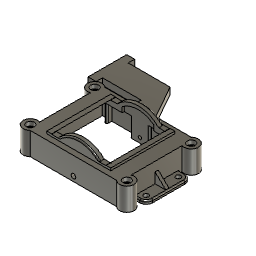
039422-01 MH Roller Assembly Top (Autodesk Fusion 360 archive; units mm, degrees)
design "039422-01 MH Roller Assembly Top" references "039423-01 MH Roller Assembly Bottom"
Autodesk Fusion 360 part; units mm, degrees
note: some values were not read from the file. Set by a fixed rule: which face or edge a step refers to.
(part 1 of 2)
derive "JointPlane" from "039423-01 MH Roller Assembly Bottom v10"
sketch "sketch 195" plane through (0, 0, 0) normal (0, 0, 1) x (1, 0, 0)
  line L0 (42.1069, 33.6931) -> (-42.1068, 33.6931)
  line L1 (-42.1068, 33.6931) -> (-42.1068, -33.6931)
  line L2 (-42.1068, -33.6931) -> (42.1069, -33.6931)
  line L3 (42.1069, -33.6931) -> (42.1069, 33.6931)
  line L4 (42.1069, 33.6931) -> (-42.1068, -33.6931) construction
  line L5 (-42.1068, 33.6931) -> (42.1069, -33.6931) construction
  line L6 (-45.2569, 36.8431) -> (45.2569, 36.8431)
  line L7 (45.2569, 36.8431) -> (45.2569, -36.8431)
  line L8 (45.2569, -36.8431) -> (-45.2569, -36.8431)
  line L9 (-45.2569, -36.8431) -> (-45.2569, 36.8431)
  line L10 (0, 36.8431) -> (0, 33.6931) construction
  line L11 (-42.1068, 0) -> (-45.2569, 0) construction
  line L12 (42.1069, 0) -> (45.2569, 0) construction
  line L13 (0, -33.6931) -> (0, -36.8431) construction
  line L14 (-47.625, 31.75) -> (47.625, 31.75) construction
  line L15 (47.625, 31.75) -> (47.625, -31.75) construction
  line L16 (47.625, -31.75) -> (-47.625, -31.75) construction
  line L17 (-47.625, -31.75) -> (-47.625, 31.75) construction
  line L18 (-47.625, 0) -> (-45.2569, 0) construction
  line L19 (47.625, 0) -> (45.2569, 0) construction
  line L20 (0, 31.75) -> (0, 33.6931) construction
  line L21 (0, -31.75) -> (0, -33.6931) construction
  circle A0 centre (47.625, -31.75) radius 2.7781
  circle A1 centre (47.625, 31.75) radius 2.7781
  circle A2 centre (-47.625, 31.75) radius 2.7781
  circle A3 centre (-47.625, -31.75) radius 2.7781
  circle A4 centre (-47.625, -31.75) radius 3.9688
  circle A5 centre (47.625, -31.75) radius 3.9688
  circle A6 centre (47.625, 31.75) radius 3.9688
  circle A7 centre (-47.625, 31.75) radius 3.9688
  circle A8 centre (-47.625, 31.75) radius 7.1188
  circle A9 centre (-47.625, -31.75) radius 7.1188
  circle A10 centre (47.625, -31.75) radius 7.1188
  circle A11 centre (47.625, 31.75) radius 7.1188
  line L22 (50.8, 15.875) -> (-50.8, 15.875) construction
  line L23 (-50.8, 15.875) -> (-50.8, -15.875) construction
  line L24 (-50.8, -15.875) -> (50.8, -15.875) construction
  line L25 (50.8, -15.875) -> (50.8, 15.875) construction
  line L26 (50.8, 15.875) -> (-50.8, -15.875) construction
  line L27 (-50.8, 15.875) -> (50.8, -15.875) construction
  circle A12 centre (-50.8, -15.875) radius 1.9558
  circle A13 centre (-50.8, 15.875) radius 1.9558
  circle A14 centre (50.8, 15.875) radius 1.9558
  circle A15 centre (50.8, -15.875) radius 1.9558
  circle A16 centre (50.8, 15.875) radius 6.35
  circle A17 centre (50.8, -15.875) radius 6.35
  circle A18 centre (-50.8, -15.875) radius 6.35
  circle A19 centre (-50.8, 15.875) radius 6.35
  line L28 (57.15, 15.875) -> (57.15, -15.875)
  line L29 (-57.15, 15.875) -> (-57.15, -15.875)
  line L30 (-50.8, -22.225) -> (-45.2569, -22.225)
  line L31 (-50.8, 22.225) -> (-45.2569, 22.225)
  line L32 (50.8, 22.225) -> (45.2569, 22.225)
  line L33 (50.8, -22.225) -> (45.2569, -22.225)
  line L34 (-45.2569, 9.525) -> (-50.8, 9.525)
  line L35 (-50.8, -9.525) -> (-45.2569, -9.525)
  line L36 (50.8, 9.525) -> (45.2569, 9.525)
  line L37 (50.8, -9.525) -> (45.2569, -9.525)
  line L38 (-42.1068, -33.6931) -> (-23.3109, -33.6931)
  line L39 (-23.3109, -33.6931) -> (-23.3109, -28.5337)
  line L40 (-23.3109, -28.5337) -> (-42.1068, -28.5337)
  line L41 (-42.1068, -28.5337) -> (-42.1068, -33.6931)
  line L42 (42.1069, -33.6931) -> (23.3109, -33.6931)
  line L43 (23.3109, -33.6931) -> (23.3109, -28.5337)
  line L44 (23.3109, -28.5337) -> (42.1069, -28.5337)
  line L45 (42.1069, -28.5337) -> (42.1069, -33.6931)
  line L46 (42.1069, 33.6931) -> (23.3109, 33.6931)
  line L47 (23.3109, 33.6931) -> (23.3109, 28.5337)
  line L48 (23.3109, 28.5337) -> (42.1069, 28.5337)
  line L49 (42.1069, 28.5337) -> (42.1069, 33.6931)
  line L50 (-42.1068, 33.6931) -> (-23.3108, 33.6931)
  line L51 (-23.3108, 33.6931) -> (-23.3108, 28.5337)
  line L52 (-23.3108, 28.5337) -> (-42.1068, 28.5337)
  line L53 (-42.1068, 28.5337) -> (-42.1068, 33.6931)
extrude "Extrude1" add sketch "sketch 195" along normal blind 22.4155 contours L0 L6 A8 A11 L46 L50 | L0 L3 L6 L7 A6 A11 L46 L49 | L0 L1 L6 L9 A7 A8 L50 L53 | L6 L7 A6 A11 | L6 L9 A7 A8 | L3 L7 A10 A11 A16 A17 | L1 L9 A8 A9 A18 A19 | L7 A1 A6 | L7 A1 A6 | L2 L3 L7 L8 A5 A10 L42 L45 | L9 A2 A7 | L9 A2 A7 | L1 L2 L8 L9 A4 A9 L38 L41 | L7 L8 A5 A10 | L9 A19 | L8 L9 A4 A9 | L7 A16 | L7 A0 A5 | L7 A0 A5 | L2 L8 A9 A10 L38 L42 | L9 A3 A4 | L9 A3 A4 | L7 A17 | L9 A18 picked at (-45.1406, 16.6644) picked at (45.1266, 16.6286) picked at (45.1266, -16.6286) picked at (-45.1406, -16.6644) makes body 1
extrude "Extrude2" add sketch "sketch 195" along normal blind 3.15 contours L9 A19 L31 | L7 A16 L32 | L9 A19 | L7 A16 | L7 A17 L33 | L9 A19 L34 | L9 A18 A19 L29 L34 L35 | L9 A18 L30 | L7 A16 L36 | L7 A16 A17 L28 L36 L37 | L7 A17 | L9 A18 | L7 A17 L37 | L9 A18 L35 picked at (-46.4526, 15.875) picked at (46.4526, 15.875) picked at (46.4526, -15.875) picked at (-46.4526, -15.875) bodies 1
sketch "sketch 867" plane through (0, 0, -3.15) normal (0, 0, -1) x (1, 0, 0)
  line L0 (-57.15, 15.875) -> (-57.15, -15.875)
  arc A0 (-50.8, -9.525) -> (-57.15, -15.875) centre (-50.8, -15.875) ccw
  line L1 (-50.8, -9.525) -> (-45.2569, -9.525)
  line L2 (-45.2569, -9.525) -> (-45.2569, 9.525)
  line L3 (-45.2569, 9.525) -> (-50.8, 9.525)
  arc A1 (-57.15, 15.875) -> (-50.8, 9.525) centre (-50.8, 15.875) ccw
  line L4 (-45.2569, 0) -> (-55.8038, 0) construction
  line L5 (-55.8038, -1.575) -> (-45.2569, -1.575)
  line L6 (-45.2569, -1.575) -> (-45.2569, 1.575)
  line L7 (-45.2569, 1.575) -> (-55.8038, 1.575)
  line L8 (-55.8038, 1.575) -> (-55.8038, -1.575)
  line L9 (-55.8038, -1.575) -> (-45.2569, 1.575) construction
  line L10 (-45.2569, -1.575) -> (-55.8038, 1.575) construction
  line L11 (45.2569, -9.525) -> (50.8, -9.525)
  arc A2 (50.8, -9.525) -> (57.15, -15.875) centre (50.8, -15.875) cw
  line L12 (57.15, -15.875) -> (57.15, 15.875)
  arc A3 (57.15, 15.875) -> (50.8, 9.525) centre (50.8, 15.875) cw
  line L13 (50.8, 9.525) -> (45.2569, 9.525)
  line L14 (45.2569, 9.525) -> (45.2569, -9.525)
  line L15 (45.2569, 0) -> (50.5303, 0) construction
  line L16 (55.8038, 1.575) -> (45.2569, 1.575)
  line L17 (45.2569, 1.575) -> (45.2569, -1.575)
  line L18 (45.2569, -1.575) -> (55.8038, -1.575)
  line L19 (55.8038, -1.575) -> (55.8038, 1.575)
  line L20 (55.8038, 1.575) -> (45.2569, -1.575) construction
  line L21 (45.2569, 1.575) -> (55.8038, -1.575) construction
extrude "Extrude3" add sketch "sketch 867" against normal blind 10.2362 from surface at -6.3 contours L2 L5 L6 L7 L8 | L14 L16 L17 L18 L19 bodies 1
sketch "OutsideSupports" plane through (0, -1.575, 0) normal (0, -1, 0) x (1, 0, 0)
  line L0 (-45.2569, 13.3862) -> (-55.8038, 13.3862)
  line L1 (-55.8038, 13.3862) -> (-55.8038, 3.15)
  line L2 (45.2568, 3.15) -> (55.8038, 3.15)
  line L3 (55.8038, 3.15) -> (55.8038, 13.3862)
  line L4 (55.8038, 13.3862) -> (45.2568, 13.3862)
  line L5 (45.2568, 13.3862) -> (45.2568, 3.15)
  line L6 (45.2568, 13.3862) -> (55.8038, 3.15)
  line L7 (-45.2569, 13.3862) -> (-55.8038, 3.15)
  line L8 (-55.8038, 3.15) -> (-45.2569, 3.15)
  line L9 (-45.2569, 3.15) -> (-45.2569, 13.3862)
  constraint coincident L4.end L5.start
  constraint coincident L2.end L3.start
  constraint coincident L0.start L7.start
  constraint coincident L1.end L7.end
extrude "Extrude4" cut sketch "OutsideSupports" against normal up to surface (3.15 mm away) contours L0 L1 L7 | L3 L4 L6 bodies 1
sketch "TopPlane" plane through (0, 0, 22.4155) normal (0, 0, 1) x (-1, 0, 0)
  line L0 (42.1068, 33.6931) -> (42.1068, -33.6931)
  line L1 (42.1068, -33.6931) -> (-42.1069, -33.6931)
  line L2 (-42.1069, -33.6931) -> (-42.1069, 33.6931)
  line L3 (-42.1069, 33.6931) -> (42.1069, 33.6931)
  arc A0 (-42.6514, 36.8431) -> (-45.2569, 25.0367) centre (-47.625, 31.75) ccw
  line L4 (-45.2569, 25.0367) -> (-45.2569, -25.0367)
  arc A1 (-45.2569, -25.0367) -> (-42.6514, -36.8431) centre (-47.625, -31.75) ccw
  line L5 (-42.6514, -36.8431) -> (42.6514, -36.8431)
  arc A2 (42.6514, -36.8431) -> (45.2569, -25.0367) centre (47.625, -31.75) ccw
  line L6 (45.2569, -25.0367) -> (45.2569, 25.0367)
  arc A3 (45.2569, 25.0367) -> (42.6514, 36.8431) centre (47.625, 31.75) ccw
  line L7 (42.6514, 36.8431) -> (-42.6514, 36.8431)
  line L8 (42.1068, -33.6931) -> (-42.1069, -33.6931)
  line L9 (-42.1069, -33.6931) -> (-42.1069, 33.6931)
  line L10 (-42.1069, 33.6931) -> (42.1068, 33.6931)
  line L11 (42.1068, 33.6931) -> (42.1068, -33.6931)
  line L12 (-26.797, -26.797) -> (26.797, -26.797)
  line L13 (26.797, -26.797) -> (26.797, 26.797)
  line L14 (26.797, 26.797) -> (-26.797, 26.797)
  line L15 (-26.797, 26.797) -> (-26.797, -26.797)
  line L16 (-26.797, -26.797) -> (26.797, 26.797) construction
  line L17 (26.797, -26.797) -> (-26.797, 26.797) construction
  line L18 (31.5595, -31.5595) -> (-31.5595, -31.5595)
  line L19 (-31.5595, -31.5595) -> (-31.5595, 31.5595)
  line L20 (-31.5595, 31.5595) -> (31.5595, 31.5595)
  line L21 (31.5595, 31.5595) -> (31.5595, -31.5595)
  line L22 (31.5595, 0) -> (26.797, 0) construction
  line L23 (-26.797, 0) -> (-31.5595, 0) construction
  line L24 (0, -26.797) -> (0, -31.5595) construction
  line L25 (0, 26.797) -> (0, 31.5595) construction
  line L26 (26.797, -26.797) -> (26.797, -31.5595)
  line L27 (-26.797, -26.797) -> (-26.797, -31.5595)
  line L28 (-26.797, 26.797) -> (-26.797, 31.5595)
  line L29 (26.797, 26.797) -> (26.797, 31.5595)
  circle A4 centre (47.625, 31.75) radius 2.7781
  circle A5 centre (47.625, -31.75) radius 2.7781
  circle A6 centre (-47.625, 31.75) radius 2.7781
  circle A7 centre (-47.625, -31.75) radius 2.7781
  circle A8 centre (-47.625, 31.75) radius 3.937
  circle A9 centre (47.625, 31.75) radius 3.937
  circle A10 centre (47.625, -31.75) radius 3.937
  circle A11 centre (-47.625, -31.75) radius 3.937
  dimension "d59" = 53.594
  dimension "d60" = 53.594
  dimension "d62" = 4.7625
  dimension "d120" = 7.874
  constraint horizontal L8
  constraint vertical L9
  constraint horizontal L10
  constraint vertical L11
  constraint coincident L2.end L3.start
  constraint coincident L0.end L1.start
  constraint horizontal L12
  constraint perpendicular L12 L13
  constraint parallel L12 L14
  constraint parallel L13 L15
  constraint coincident L16 origin
  constraint coincident L17 origin
  constraint horizontal L18
  constraint vertical L19
  constraint horizontal L20
  constraint vertical L21
  constraint midpoint L21 L22.start
  constraint midpoint L13 L22.end
  constraint midpoint L15 L23.start
  constraint midpoint L19 L23.end
  constraint midpoint L12 L24.start
  constraint midpoint L18 L24.end
  constraint midpoint L14 L25.start
  constraint midpoint L20 L25.end
  constraint equal L22 L24
  constraint vertical L24
  constraint horizontal L22
  constraint coincident L18 L26.end
  constraint perpendicular L18 L26
  constraint coincident L18 L27.end
  constraint perpendicular L18 L27
  constraint coincident L20 L28.end
  constraint perpendicular L20 L28
  constraint coincident L20 L29.end
  constraint perpendicular L20 L29
  constraint concentric A0 A8
  constraint concentric A3 A9
  constraint concentric A2 A10
  constraint concentric A1 A11
  constraint equal A8 A9
  constraint equal A9 A10
  constraint equal A10 A11
  measures "d59" distance of L12.end L13.end
  measures "d60" distance of L12.start L12.end
  measures "d62" distance of L22.start L22.end
  measures "d120" diameter of A8
extrude "Extrude5" add sketch "TopPlane" against normal blind 3.15 contours L0 L1 L2 L3 L8 L9 L10 L11 | L15 L18 L19 L20 L27 L28 | L12 L18 L26 L27 | L13 L18 L20 L21 L26 L29 | L14 L20 L28 L29 bodies 1
extrude "Extrude6" add sketch "TopPlane" along normal blind 2.3813 contours L15 L18 L19 L20 L27 L28 | L13 L18 L20 L21 L26 L29 bodies 1
fillet "Fillet1" radius 1.27 5 edges at (48.0284, -22.225, 3.15) (55.2901, -20.3651, 3.15) (57.15, 0, 3.15) (55.2901, 20.3651, 3.15) (48.0284, 22.225, 3.15) on bodies 1
fillet "Fillet1" radius 1.27 5 edges at (-48.0284, 22.225, 3.15) (-55.2901, 20.3651, 3.15) (-57.15, 0, 3.15) (-55.2901, -20.3651, 3.15) (-48.0284, -22.225, 3.15) on bodies 1
extrude "Extrude7" add sketch "TopPlane" along normal blind 1.9844 contours L12 L18 L26 L27 | L14 L20 L28 L29 bodies 1
sketch "FrontOuterPegHole" plane through (0, -36.8431, 0) normal (0, -1, 0) x (1, 0, 0)
  line L0 (-42.6514, 0) -> (42.6514, 0)
  line L1 (42.6514, 0) -> (42.6514, 22.4155)
  line L2 (42.6514, 22.4155) -> (-42.6514, 22.4155)
  line L3 (-42.6514, 22.4155) -> (-42.6514, 0)
  line L4 (0, 0) -> (0, 4.7244) construction
  circle A0 centre (0, 4.7244) radius 2.3241
  dimension "d76" = 4.6482
  dimension "d78" = 4.7244
  constraint coincident L4.start origin
  constraint perpendicular L0 L4
  constraint coincident L4.end A0.centre
  measures "d76" diameter of A0
  measures "d78" distance of L4.start L4.end
sketch "PinchGuardReferenceCircle" plane through (0, -31.5595, 0) normal (0, -1, 0) x (1, 0, 0)
  line L0 (-31.5595, 22.4155) -> (31.5595, 22.4155)
  line L1 (31.5595, 22.4155) -> (31.5595, 24.7967)
  line L2 (31.5595, 24.7967) -> (26.797, 24.7967)
  line L3 (26.797, 24.7967) -> (26.797, 24.3999)
  line L4 (26.797, 24.3999) -> (-26.797, 24.3999)
  line L5 (-26.797, 24.3999) -> (-26.797, 24.7967)
  line L6 (-26.797, 24.7967) -> (-31.5595, 24.7967)
  line L7 (-31.5595, 24.7967) -> (-31.5595, 22.4155)
  circle A0 centre (0, 4.7244) radius 28.3591
  point P0 (0, 4.7244)
  dimension "d80" = 56.7182
  constraint coincident P0 A0.centre
  measures "d80" diameter of A0
extrude "Extrude8" add sketch "PinchGuardReferenceCircle" against normal up to surface (4.7625 mm away) contours L4 A0 bodies 1
extrude "Extrude9" add sketch "PinchGuardReferenceCircle" against normal up to surface (4.7625 mm away) from surface at -58.3565 contours L4 A0 bodies 1
fillet "Fillet2" radius 1.27 2 edges at (0, 31.5595, 33.0835) (0, -31.5595, 33.0835) on bodies 1
sketch "RearInnerPinchGuard" plane through (0, 26.797, 0) normal (0, -1, 0) x (1, 0, 0)
  line L0 (-26.797, 24.3999) -> (-26.797, 19.2655)
  line L1 (-26.797, 19.2655) -> (26.797, 19.2655)
  line L2 (26.797, 19.2655) -> (26.797, 24.3999)
  line L3 (26.797, 24.3999) -> (20.4234, 24.3999)
  arc A0 (20.4234, 24.3999) -> (-20.4234, 24.3999) centre (0, 4.7244) ccw
  line L4 (-20.4234, 24.3999) -> (-26.797, 24.3999)
  circle A1 centre (0, 4.7244) radius 25.1206
  circle A2 centre (0, 4.7244) radius 28.3591
  line L5 (26.797, 24.3999) -> (-26.797, 24.3999)
  line L6 (-15.6179, 24.3999) -> (-15.6179, 19.2655)
  line L7 (15.6179, 24.3999) -> (15.6179, 19.2655)
  line L8 (-15.6179, 19.2655) -> (15.6179, 19.2655)
  point P0 (-15.6179, 24.3999)
  point P1 (15.6179, 24.3999)
  dimension "d90" = 3.2385
  constraint concentric A0 A1
  constraint coincident A1 P0
  constraint coincident P0 L5
  constraint coincident A1 P1
  constraint coincident L5 P1
  constraint coincident P0 L6.start
  constraint coincident L1 L6.end
  constraint perpendicular L1 L6
  constraint coincident P1 L7.start
  constraint coincident L1 L7.end
  constraint perpendicular L1 L7
  measures "d90" distance of A1 A2
sketch "FrontInnerPinchGuard" plane through (0, -26.797, 0) normal (0, 1, 0) x (-1, 0, 0)
  line L0 (-26.797, 24.3999) -> (-26.797, 19.2655)
  line L1 (-26.797, 19.2655) -> (26.797, 19.2655)
  line L2 (26.797, 19.2655) -> (26.797, 24.3999)
  line L3 (26.797, 24.3999) -> (20.4234, 24.3999)
  arc A0 (20.4234, 24.3999) -> (-20.4234, 24.3999) centre (0, 4.7244) ccw
  line L4 (-20.4234, 24.3999) -> (-26.797, 24.3999)
  circle A1 centre (0, 4.7244) radius 25.1206
  line L5 (-15.6179, 24.3999) -> (-15.6179, 19.2655)
  line L6 (15.6179, 24.3999) -> (15.6179, 19.2655)
  line L7 (15.6179, 19.2655) -> (-15.6179, 19.2655)
extrude "Extrude10" cut sketch "FrontInnerPinchGuard" against normal blind 1.9844 contours L1 A1 L5 L6 L7 bodies 1
extrude "Extrude11" cut sketch "RearInnerPinchGuard" against normal blind 1.9844 contours A1 L5 | L1 L5 L6 L7 L8 bodies 1
sketch "PegFlapsAndInnerSupportBase" plane through (0, 0, 19.2655) normal (0, 0, -1) x (1, 0, 0)
  line L0 (15.6179, -26.797) -> (15.6179, -28.7814)
  line L1 (15.6179, -28.7814) -> (-15.6179, -28.7814)
  line L2 (-15.6179, -28.7814) -> (-15.6179, -26.797)
  line L3 (-15.6179, -26.797) -> (-26.797, -26.797)
  line L4 (-26.797, -26.797) -> (-26.797, 26.797)
  line L5 (-26.797, 26.797) -> (-15.6179, 26.797)
  line L6 (-15.6179, 26.797) -> (-15.6179, 28.7814)
  line L7 (-15.6179, 28.7814) -> (15.6179, 28.7814)
  line L8 (15.6179, 28.7814) -> (15.6179, 26.797)
  line L9 (15.6179, 26.797) -> (26.797, 26.797)
  line L10 (26.797, 26.797) -> (26.797, -26.797)
  line L11 (26.797, -26.797) -> (15.6179, -26.797)
  line L12 (42.1069, 33.6931) -> (-42.1068, 33.6931)
  line L13 (-42.1068, 33.6931) -> (-42.1068, -33.6931)
  line L14 (-42.1068, -33.6931) -> (42.1069, -33.6931)
  line L15 (42.1069, -33.6931) -> (42.1069, 33.6931)
  line L16 (-9.525, -31.9564) -> (9.525, -31.9564)
  line L17 (9.525, -31.9564) -> (9.525, -28.7814)
  line L18 (9.525, -28.7814) -> (-9.525, -28.7814)
  line L19 (-9.525, -28.7814) -> (-9.525, -31.9564)
  line L20 (-9.525, -31.9564) -> (9.525, -28.7814) construction
  line L21 (9.525, -31.9564) -> (-9.525, -28.7814) construction
  line L22 (0, -30.3689) -> (0, 0) construction
  line L23 (-9.525, 28.7814) -> (-9.525, 31.9564)
  line L24 (0, 30.3689) -> (0, 0) construction
  line L25 (9.525, 28.7814) -> (-9.525, 31.9564) construction
  line L26 (9.525, 31.9564) -> (9.525, 28.7814)
  line L27 (9.525, 28.7814) -> (-9.525, 28.7814)
  line L28 (-9.525, 31.9564) -> (9.525, 31.9564)
  line L29 (-9.525, 28.7814) -> (9.525, 31.9564) construction
  line L30 (-50.8, 15.875) -> (50.8, 15.875) construction
  line L31 (50.8, -15.875) -> (-50.8, -15.875) construction
  line L32 (-26.797, 17.45) -> (-42.1068, 17.45)
  line L33 (-42.1068, 17.45) -> (-42.1068, 14.3)
  line L34 (-42.1068, 14.3) -> (-26.797, 14.3)
  line L35 (-26.797, 14.3) -> (-26.797, 17.45)
  line L36 (-26.797, 17.45) -> (-42.1068, 14.3) construction
  line L37 (-42.1068, 17.45) -> (-26.797, 14.3) construction
  line L38 (42.1069, 17.45) -> (26.797, 17.45)
  line L39 (26.797, 17.45) -> (26.797, 14.3)
  line L40 (26.797, 14.3) -> (42.1069, 14.3)
  line L41 (42.1069, 14.3) -> (42.1069, 17.45)
  line L42 (42.1069, 17.45) -> (26.797, 14.3) construction
  line L43 (26.797, 17.45) -> (42.1069, 14.3) construction
  line L44 (-42.1068, -33.6931) -> (-42.1068, 33.6931)
  line L45 (-26.797, -26.797) -> (-26.797, 26.797)
  line L46 (42.1069, 33.6931) -> (42.1069, -33.6931)
  line L47 (26.797, 26.797) -> (26.797, -26.797)
  line L48 (-26.797, -14.3) -> (-42.1068, -14.3)
  line L49 (-42.1068, -14.3) -> (-42.1068, -17.45)
  line L50 (-42.1068, -17.45) -> (-26.797, -17.45)
  line L51 (-26.797, -17.45) -> (-26.797, -14.3)
  line L52 (-26.797, -14.3) -> (-42.1068, -17.45) construction
  line L53 (-42.1068, -14.3) -> (-26.797, -17.45) construction
  line L54 (26.797, -14.3) -> (42.1069, -14.3)
  line L55 (42.1069, -14.3) -> (42.1069, -17.45)
  line L56 (42.1069, -17.45) -> (26.797, -17.45)
  line L57 (26.797, -17.45) -> (26.797, -14.3)
  line L58 (26.797, -14.3) -> (42.1069, -17.45) construction
  line L59 (42.1069, -14.3) -> (26.797, -17.45) construction
  line L60 (-35.7568, -33.6931) -> (-32.6068, -33.6931)
  line L61 (-32.6068, -33.6931) -> (-32.6068, -28.9306)
  line L62 (-32.6068, -28.9306) -> (-35.7568, -28.9306)
  line L63 (-35.7568, -28.9306) -> (-35.7568, -33.6931)
  line L64 (32.6069, -33.6931) -> (35.7569, -33.6931)
  line L65 (35.7569, -33.6931) -> (35.7569, -28.9306)
  line L66 (35.7569, -28.9306) -> (32.6069, -28.9306)
  line L67 (32.6069, -28.9306) -> (32.6069, -33.6931)
  line L68 (35.7569, 33.6931) -> (32.6069, 33.6931)
  line L69 (32.6069, 33.6931) -> (32.6069, 28.9306)
  line L70 (32.6069, 28.9306) -> (35.7569, 28.9306)
  line L71 (35.7569, 28.9306) -> (35.7569, 33.6931)
  line L72 (-32.6068, 33.6931) -> (-35.7568, 33.6931)
  line L73 (-35.7568, 33.6931) -> (-35.7568, 28.9306)
  line L74 (-35.7568, 28.9306) -> (-32.6068, 28.9306)
  line L75 (-32.6068, 28.9306) -> (-32.6068, 33.6931)
  line L76 (42.1069, -33.6931) -> (35.7569, -33.6931) construction
  line L77 (-35.7568, -33.6931) -> (-42.1068, -33.6931) construction
  line L78 (-35.7568, 33.6931) -> (-42.1068, 33.6931) construction
  line L79 (35.7569, 33.6931) -> (42.1069, 33.6931) construction
  point P0 (0, -30.3689)
  point P1 (0, 30.3689)
  point P2 (-34.4519, 15.875)
  point P3 (34.4519, 15.875)
  point P4 (-34.4519, -15.875)
  point P5 (34.4519, -15.875)
  dimension "d98" = 19.05
  dimension "d99" = 3.175
  dimension "d100" = 19.05
  dimension "d101" = 3.175
  dimension "d123" = 3.15
  dimension "d148" = 3.15
  dimension "d149" = 3.15
  dimension "d150" = 3.15
  dimension "d151" = 3.15
  dimension "d153" = 4.7625
  dimension "d154" = 6.35
  constraint horizontal L16
  constraint perpendicular L16 L17
  constraint parallel L16 L18
  constraint parallel L17 L19
  constraint coincident L20 P0
  constraint coincident L21 P0
  constraint coincident P0 L22.start
  constraint coincident L22.end L24.end
  constraint vertical L22
  constraint collinear L1 L18
  constraint perpendicular L23 L27
  constraint parallel L27 L28
  constraint parallel L23 L26
  constraint coincident P1 L25
  constraint coincident P1 L29
  constraint coincident P1 L24.start
  constraint collinear L7 L27
  constraint vertical L24
  constraint horizontal L32
  constraint perpendicular L32 L33
  constraint parallel L32 L34
  constraint parallel L33 L35
  constraint coincident L36 P2
  constraint coincident L37 P2
  constraint coincident L30 P2
  constraint horizontal L38
  constraint perpendicular L38 L39
  constraint parallel L38 L40
  constraint parallel L39 L41
  constraint coincident L42 P3
  constraint coincident L43 P3
  constraint coincident L30 P3
  constraint collinear L33 L44
  constraint collinear L35 L45
  constraint collinear L41 L46
  constraint collinear L39 L47
  constraint equal L35 L39
  constraint horizontal L48
  constraint perpendicular L48 L49
  constraint parallel L48 L50
  constraint parallel L49 L51
  constraint coincident L52 P4
  constraint coincident L53 P4
  constraint coincident L31 P4
  constraint horizontal L54
  constraint perpendicular L54 L55
  constraint parallel L54 L56
  constraint parallel L55 L57
  constraint coincident L58 P5
  constraint coincident L59 P5
  constraint coincident L31 P5
  constraint equal L51 L57
  constraint equal L35 L51
  constraint collinear L44 L49
  constraint collinear L45 L51
  constraint collinear L46 L55
  constraint collinear L47 L57
  constraint horizontal L60
  constraint vertical L61
  constraint horizontal L62
  constraint vertical L63
  constraint coincident L14 L60.start
  constraint horizontal L64
  constraint vertical L65
  constraint horizontal L66
  constraint vertical L67
  constraint coincident L14 L64.start
  constraint horizontal L68
  constraint vertical L69
  constraint horizontal L70
  constraint vertical L71
  constraint coincident L12 L68.start
  constraint horizontal L72
  constraint vertical L73
  constraint horizontal L74
  constraint vertical L75
  constraint coincident L12 L72.start
  constraint equal L69 L73
  constraint equal L67 L69
  constraint equal L63 L67
  constraint coincident L14.end L15.start
  constraint coincident L13.end L14.start
  constraint perpendicular L13 L77
  constraint coincident L12.end L13.start
  constraint perpendicular L13 L78
  constraint coincident L12.start L15.end
  constraint perpendicular L46 L79
  constraint equal L78 L79
  constraint equal L76 L79
  constraint equal L76 L77
  measures "d98" distance of L17.end L18.end
  measures "d99" distance of L16.start L18.end
  measures "d100" distance of L26.start L23.end
  measures "d101" distance of L25.start L26.start
  measures "d123" distance of L32.start L34.end
  measures "d148" distance of L60.start L60.end
  measures "d149" distance of L64.start L64.end
  measures "d150" distance of L68.start L68.end
  measures "d151" distance of L72.start L72.end
  measures "d153" distance of L72.end L73.end
  measures "d154" distance of L60.start L13.end
extrude "Extrude12" add sketch "PegFlapsAndInnerSupportBase" along normal up to surface (19.2655 mm away) contours L1 L16 L17 L18 L19 | L14 L64 L65 L66 L67 | L14 L60 L61 L62 L63 | L12 L68 L69 L70 L71 | L7 L23 L26 L27 L28 | L12 L72 L73 L74 L75 bodies 1
fillet "Fillet3" radius 1.27 8 edges at (-9.525, 28.7814, 9.6327) (-9.525, 31.9564, 9.6327) (9.525, 28.7814, 9.6327) (-9.525, -31.9564, 9.6327) (-9.525, -28.7814, 9.6327) (9.525, -31.9564, 9.6327) (9.525, -28.7814, 9.6327) (9.525, 31.9564, 9.6327) on bodies 1
fillet "Fillet3" radius 1.27 8 edges at (-35.7568, -28.9306, 9.6327) (-32.6068, -28.9306, 9.6327) (32.6069, -28.9306, 9.6327) (35.7569, -28.9306, 9.6327) (-35.7568, 28.9306, 9.6327) (-32.6068, 28.9306, 9.6327) (32.6069, 28.9306, 9.6327) (35.7569, 28.9306, 9.6327) on bodies 1
sketch "RearOuterPegHole" plane through (0, 36.8431, 0) normal (0, 1, 0) x (-1, 0, 0)
  line L0 (-42.6514, 0) -> (42.6514, 0)
  line L1 (42.6514, 0) -> (42.6514, 22.4155)
  line L2 (42.6514, 22.4155) -> (-42.6514, 22.4155)
  line L3 (-42.6514, 22.4155) -> (-42.6514, 0)
  circle A0 centre (0, 4.7244) radius 2.3241
  circle A1 centre (0, 4.7244) radius 2.3241
  point P0 (0, 4.7244)
  constraint concentric A0 A1
  constraint equal A0 A1
extrude "Extrude13" cut sketch "RearOuterPegHole" against normal up to surface (3.15 mm away) contours A0 A1 bodies 1
extrude "Extrude14" cut sketch "FrontOuterPegHole" against normal up to surface (3.15 mm away) contours A0 bodies 1
sketch "InnerPegHoles" plane through (0, -31.9564, 0) normal (0, -1, 0) x (1, 0, 0)
  line L0 (8.255, 0) -> (8.255, 19.2655)
  line L1 (8.255, 19.2655) -> (-8.255, 19.2655)
  line L2 (-8.255, 19.2655) -> (-8.255, 0)
  line L3 (-8.255, 0) -> (8.255, 0)
  circle A0 centre (0, 4.7244) radius 1.632
  point P0 (0, 4.7244)
  dimension "d111" = 3.2639
  constraint coincident P0 A0.centre
  measures "d111" diameter of A0
extrude "Extrude15" cut sketch "InnerPegHoles" against normal up to surface (63.9127 mm away) contours A0 bodies 1
sketch "JointCounterbores" plane through (0, 0, 0) normal (0, 0, -1) x (1, 0, 0)
  circle A0 centre (50.8, 15.875) radius 1.9558
  circle A1 centre (50.8, -15.875) radius 1.9558
  circle A2 centre (-50.8, 15.875) radius 1.9558
  circle A3 centre (-50.8, -15.875) radius 1.9558
  circle A4 centre (-47.625, 31.75) radius 2.7781
  circle A5 centre (-47.625, -31.75) radius 2.7781
  line L0 (-42.1068, -33.6931) -> (-42.1068, 33.6931)
  line L1 (-42.1068, 33.6931) -> (-35.7568, 33.6931)
  line L2 (42.1069, 33.6931) -> (42.1069, -33.6931)
  line L3 (42.1069, -33.6931) -> (35.7569, -33.6931)
  circle A6 centre (47.625, 31.75) radius 2.7781
  circle A7 centre (47.625, -31.75) radius 2.7781
  arc A8 (45.2569, 25.0367) -> (42.6514, 36.8431) centre (47.625, 31.75) ccw
  line L4 (42.6514, 36.8431) -> (-42.6514, 36.8431)
  arc A9 (-42.6514, 36.8431) -> (-45.2569, 25.0367) centre (-47.625, 31.75) ccw
  line L5 (-45.2569, 25.0367) -> (-45.2569, 22.225)
  line L6 (-45.2569, 22.225) -> (-50.8, 22.225)
  arc A10 (-50.8, 22.225) -> (-57.15, 15.875) centre (-50.8, 15.875) ccw
  line L7 (-57.15, 15.875) -> (-57.15, -15.875)
  arc A11 (-57.15, -15.875) -> (-50.8, -22.225) centre (-50.8, -15.875) ccw
  line L8 (-50.8, -22.225) -> (-45.2569, -22.225)
  line L9 (-45.2569, -22.225) -> (-45.2569, -25.0367)
  arc A12 (-45.2569, -25.0367) -> (-42.6514, -36.8431) centre (-47.625, -31.75) ccw
  line L10 (-42.6514, -36.8431) -> (42.6514, -36.8431)
  arc A13 (42.6514, -36.8431) -> (45.2569, -25.0367) centre (47.625, -31.75) ccw
  line L11 (45.2569, -25.0367) -> (45.2569, -22.225)
  line L12 (45.2569, -22.225) -> (50.8, -22.225)
  arc A14 (50.8, -22.225) -> (57.15, -15.875) centre (50.8, -15.875) ccw
  line L13 (57.15, -15.875) -> (57.15, 15.875)
  arc A15 (57.15, 15.875) -> (50.8, 22.225) centre (50.8, 15.875) ccw
  line L14 (50.8, 22.225) -> (45.2569, 22.225)
  line L15 (45.2569, 22.225) -> (45.2569, 25.0367)
  circle A16 centre (-47.625, 31.75) radius 4.0323
  circle A17 centre (47.625, 31.75) radius 4.0323
  circle A18 centre (47.625, -31.75) radius 4.0323
  circle A19 centre (-47.625, -31.75) radius 4.0323
  line L16 (-35.7568, 33.6931) -> (-35.7568, 30.2006)
  line L17 (-34.4868, 28.9306) -> (-33.8768, 28.9306)
  line L18 (-32.6068, 30.2006) -> (-32.6068, 33.6931)
  line L19 (-32.6068, 33.6931) -> (32.6069, 33.6931)
  line L20 (32.6069, 33.6931) -> (32.6069, 30.2006)
  line L21 (33.8769, 28.9306) -> (34.4869, 28.9306)
  line L22 (35.7569, 30.2006) -> (35.7569, 33.6931)
  line L23 (35.7569, 33.6931) -> (42.1069, 33.6931)
  line L24 (35.7569, -33.6931) -> (35.7569, -30.2006)
  line L25 (34.4869, -28.9306) -> (33.8769, -28.9306)
  line L26 (32.6069, -30.2006) -> (32.6069, -33.6931)
  line L27 (32.6069, -33.6931) -> (-32.6068, -33.6931)
  line L28 (-32.6068, -33.6931) -> (-32.6068, -30.2006)
  line L29 (-33.8768, -28.9306) -> (-34.4868, -28.9306)
  line L30 (-35.7568, -30.2006) -> (-35.7568, -33.6931)
  line L31 (-35.7568, -33.6931) -> (-42.1068, -33.6931)
  arc A20 (35.7569, -30.2006) -> (34.4869, -28.9306) centre (34.4869, -30.2006) ccw
  arc A21 (33.8769, -28.9306) -> (32.6069, -30.2006) centre (33.8769, -30.2006) ccw
  arc A22 (-32.6068, -30.2006) -> (-33.8768, -28.9306) centre (-33.8768, -30.2006) ccw
  arc A23 (-34.4868, -28.9306) -> (-35.7568, -30.2006) centre (-34.4868, -30.2006) ccw
  arc A24 (-35.7569, 30.2006) -> (-34.4868, 28.9306) centre (-34.4868, 30.2006) ccw
  arc A25 (-33.8768, 28.9306) -> (-32.6068, 30.2006) centre (-33.8768, 30.2006) ccw
  arc A26 (32.6069, 30.2006) -> (33.8769, 28.9306) centre (33.8769, 30.2006) ccw
  arc A27 (34.4869, 28.9306) -> (35.7569, 30.2006) centre (34.4869, 30.2006) ccw
  dimension "d117" = 8.0645
  constraint concentric A4 A16
  constraint concentric A6 A17
  constraint concentric A7 A18
  constraint concentric A5 A19
  constraint equal A16 A17
  constraint equal A17 A18
  constraint equal A18 A19
  measures "d117" diameter of A16
extrude "Extrude16" cut sketch "JointCounterbores" against normal blind 4.064 contours A16 | A17 | A18 | A19 bodies 1
extrude "Extrude17" cut sketch "TopPlane" against normal blind 4.064 contours A8 | A9 | A10 | A11 bodies 1
extrude "Extrude18" add sketch "PegFlapsAndInnerSupportBase" along normal blind 9.7536 contours L10 L15 L46 L47 L54 L55 L56 L57 | L10 L15 L38 L39 L40 L41 L46 L47 | L4 L13 L44 L45 L48 L49 L50 L51 | L4 L13 L32 L33 L34 L35 L44 L45 bodies 1
sketch "InnerSupports" plane through (0, 17.45, 0) normal (0, 1, 0) x (-1, 0, 0)
  line L0 (42.1068, 19.2655) -> (26.797, 19.2655)
  line L1 (26.797, 19.2655) -> (26.797, 9.5119)
  line L2 (26.797, 9.5119) -> (42.1068, 9.5119)
  line L3 (42.1068, 9.5119) -> (42.1068, 19.2655)
  line L4 (-26.797, 19.2655) -> (-42.1069, 19.2655)
  line L5 (-42.1069, 19.2655) -> (-42.1069, 9.5119)
  line L6 (-42.1069, 9.5119) -> (-26.797, 9.5119)
  line L7 (-26.797, 9.5119) -> (-26.797, 19.2655)
  line L8 (-26.797, 24.7967) -> (-31.5595, 24.7967)
  line L9 (-31.5595, 24.7967) -> (-26.797, 24.7967)
  line L10 (26.797, 24.7967) -> (31.5595, 24.7967)
  line L11 (31.5595, 24.7967) -> (26.797, 24.7967)
  line L12 (-26.797, 24.7967) -> (-26.797, 9.5119)
  line L13 (26.797, 9.5119) -> (26.797, 24.7967)
  line L14 (-42.1069, 9.5119) -> (-32.9477, 19.2655)
  line L15 (-42.1069, 9.5119) -> (-35.0981, 9.5119) construction
  line L16 (42.1068, 9.5119) -> (32.9477, 19.2655)
  line L17 (42.1068, 9.5119) -> (33.1786, 9.5119) construction
  line L18 (26.797, 24.7967) -> (42.1068, 9.9564)
  line L19 (-26.797, 24.7967) -> (-42.1069, 9.9564)
  line L20 (42.1068, 9.5119) -> (42.1068, 9.9564) construction
  line L21 (32.9477, 19.2655) -> (32.5032, 19.2655) construction
  line L22 (-42.1069, 9.5119) -> (-42.1069, 9.9564) construction
  line L23 (-32.9477, 19.2655) -> (-32.5032, 19.2655) construction
  dimension "d147" = 0.4445
  constraint coincident L8.start L9.end
  constraint coincident L6.end L7.start
  constraint coincident L1.end L2.start
  constraint coincident L10.start L11.end
  constraint horizontal L15
  constraint coincident L5.end L6.start
  constraint coincident L4 L14.end
  constraint horizontal L17
  constraint coincident L2.end L3.start
  constraint coincident L0 L16.end
  constraint coincident L3 L18.end
  constraint coincident L5 L19.end
  constraint coincident L18 L21.end
  constraint coincident L0 L21.end
  constraint equal L20 L21
  constraint perpendicular L6 L22
  constraint coincident L19 L23.end
  constraint coincident L4 L23.end
  constraint equal L22 L23
  constraint equal L21 L23
  measures "d147" distance of L2.end L18.end
extrude "Extrude19" cut sketch "InnerSupports" along normal up to surface (9.347 mm away) and the other way up to surface (44.247 mm away) contours L0 L16 L18 | L0 L1 L2 L13 L16 L18 | L0 L13 L18 | L4 L14 L19 | L4 L12 L19 | L4 L6 L7 L12 L14 L19 bodies 1
ref_plane "WorkPlane1" through (-61.9125, 58.547, -33.3375) normal (1, 0, 0) x (0, 1, 0)
sketch "EncodingArmDistance" plane through (-61.9125, 0, 0) normal (1, 0, 0) x (0, 1, 0)
  line L0 (77.597, -33.3375) -> (39.497, -33.3375) construction
  line L1 (39.497, -33.3375) -> (39.497, 20.3708) construction
  line L2 (39.497, 20.3708) -> (77.597, 20.3708) construction
  line L3 (77.597, 20.3708) -> (77.597, -33.3375) construction
  point P0 (39.497, -33.3375)
  point P1 (58.547, -33.3375)
  point P2 (77.597, -33.3375)
  dimension "d132" = 53.7083
  constraint horizontal L0
  constraint vertical L1
  constraint horizontal L2
  constraint vertical L3
  constraint coincident P2 L0.start
  constraint coincident P0 L0.end
  measures "d132" distance of P2 L2.end
ref_plane "WorkPlane2" through (-61.9125, 58.547, 20.3708) normal (0, 0, 1) x (0, 1, 0)
sketch "UpperEncodingArm" plane through (0, 0, 20.3708) normal (0, 0, 1) x (1, 0, 0)
  line L0 (-12.725, 71.247) -> (6.5659, 36.8431)
  line L1 (-12.725, 65.6292) -> (3.4159, 36.8431)
  line L2 (-15.875, 71.247) -> (-53.975, 71.247)
  line L3 (-53.975, 68.097) -> (-15.875, 68.097)
  line L4 (-53.975, 48.997) -> (-15.875, 48.997)
  line L5 (-53.975, 45.847) -> (-15.875, 45.847)
  line L6 (-15.875, 45.847) -> (-15.875, 71.247)
  line L7 (-15.875, 36.8431) -> (-15.875, 71.247)
  line L8 (-12.725, 36.8431) -> (-12.725, 65.6292)
  line L9 (-53.975, 77.597) -> (-53.975, 39.497)
  line L10 (-57.1119, 74.0251) -> (-57.1119, 43.0689)
  line L11 (-58.7756, 43.0689) -> (-58.7756, 74.0251)
  line L12 (-12.725, 65.6292) -> (-12.725, 68.097)
  line L13 (-12.725, 68.097) -> (-15.875, 68.097)
  line L14 (-15.875, 71.247) -> (-12.725, 71.247)
  line L15 (-53.975, 39.497) -> (-61.9125, 39.497)
  line L16 (-61.9125, 77.597) -> (-53.975, 77.597)
  line L17 (-61.9125, 39.497) -> (-61.9125, 77.597)
  line L18 (-58.7756, 74.0251) -> (-57.1119, 74.0251)
  line L19 (-57.1119, 43.0689) -> (-58.7756, 43.0689)
  line L20 (-57.9438, 43.0689) -> (-57.9438, 39.497)
  line L21 (-57.9438, 74.0251) -> (-57.9438, 77.597)
  line L22 (-57.1119, 58.547) -> (-53.975, 58.547)
  line L23 (-58.7756, 58.547) -> (-61.9125, 58.547)
  line L24 (-47.625, 31.75) -> (-47.625, 71.247)
  line L25 (-12.725, 36.8431) -> (-15.875, 36.8431)
  line L26 (6.5659, 36.8431) -> (3.4159, 36.8431)
  line L27 (3.4159, 36.8431) -> (-12.725, 36.8431)
  constraint coincident L8.start L25.start
  constraint coincident L7.start L25.end
  constraint coincident L0.end L26.start
  constraint coincident L1.end L26.end
extrude "Extrude20" add sketch "UpperEncodingArm" against normal blind 2.9083 contours L1 L8 L27 | L3 L4 L6 L7 L24 | L3 L4 L9 L24 | L10 L11 L18 L19 bodies 1 makes body 2 at (-28.575, 55.3637, 20.3708) makes body 3 at (-57.1119, 63.7064, 19.4014)
extrude "Extrude21" add sketch "UpperEncodingArm" against normal blind 6.5532 contours L0 L1 L6 L7 L12 L13 L14 L26 | L2 L3 L6 L7 L24 | L2 L3 L9 L24 | L9 L10 L16 L18 L21 L22 | L4 L5 L6 L7 L24 | L4 L5 L9 L24 | L11 L16 L17 L18 L21 L23 | L9 L10 L15 L19 L20 L22 | L11 L15 L17 L19 L20 L23 bodies 1 2 3
extrude "Extrude22" add sketch "UpperEncodingArm" against normal blind 14.0589 contours L6 L7 L8 L12 L13 L25 bodies 1
sketch "UpperEncodingArmSupport" plane through (-15.875, 0, 0) normal (-1, 0, 0) x (0, -1, 0)
  line L0 (-45.847, 20.3708) -> (-45.847, 13.8176)
  line L1 (-45.847, 13.8176) -> (-48.997, 13.8176)
  line L2 (-48.997, 13.8176) -> (-48.997, 17.4625)
  line L3 (-48.997, 17.4625) -> (-68.097, 17.4625)
  line L4 (-68.097, 17.4625) -> (-68.097, 13.8176)
  line L5 (-68.097, 13.8176) -> (-68.097, 6.3119)
  line L6 (-68.097, 6.3119) -> (-36.8431, 6.3119)
  line L7 (-36.8431, 6.3119) -> (-36.8431, 20.3708)
  line L8 (-36.8431, 20.3708) -> (-45.847, 20.3708)
  line L9 (-71.247, 13.8176) -> (-68.097, 13.8176)
  line L10 (-48.997, 13.8176) -> (-45.847, 13.8176)
  line L11 (-36.8431, 6.3119) -> (-68.097, 13.8176)
  constraint coincident L6.end L7.start
  constraint coincident L4.end L5.start
extrude "Extrude23" cut sketch "UpperEncodingArmSupport" against normal up to surface (3.15 mm away) contours L5 L6 L11 bodies 1
sketch "Sketch16" plane through (0, 0, 3.15) normal (0, 0, 1) x (-1, 0, 0)
  line L0 (50.8, 20.955) -> (45.2569, 20.955)
  line L1 (45.2569, 20.955) -> (45.2569, 1.575)
  line L2 (45.2569, 1.575) -> (55.8038, 1.575)
  line L3 (55.8038, 1.575) -> (55.8038, -1.575)
  line L4 (55.8038, -1.575) -> (45.2569, -1.575)
  line L5 (45.2569, -1.575) -> (45.2569, -20.955)
  line L6 (45.2569, -20.955) -> (50.8, -20.955)
  arc A0 (50.8, -20.955) -> (55.88, -15.875) centre (50.8, -15.875) ccw
  line L7 (55.88, -15.875) -> (55.88, 15.875)
  arc A1 (55.88, 15.875) -> (50.8, 20.955) centre (50.8, 15.875) ccw
  circle A2 centre (50.8, -15.875) radius 1.9558
  circle A3 centre (50.8, 15.875) radius 1.9558
  circle A4 centre (50.8, 15.875) radius 1.9558
  circle A5 centre (50.8, -15.875) radius 1.9558
  circle A6 centre (-50.8, -15.875) radius 1.9558
  circle A7 centre (-50.8, 15.875) radius 1.9558
  circle A8 centre (-50.8, 15.875) radius 2.3812
  circle A9 centre (-50.8, -15.875) radius 2.3812
  circle A10 centre (50.8, 15.875) radius 2.3812
  circle A11 centre (50.8, -15.875) radius 2.3812
  dimension "d204" = 4.7625
  constraint concentric A7 A8
  constraint concentric A6 A9
  constraint concentric A4 A10
  constraint concentric A5 A11
  constraint equal A8 A9
  constraint equal A9 A11
  constraint equal A10 A11
  measures "d204" diameter of A8
extrude "Extrude24" cut sketch "Sketch16" against normal up to surface (3.15 mm away) contours A2 A5 | A3 A4 | A6 | A7 | A8 | A9 | A10 | A11 bodies 1
equation "d1 = UpperBodyHeight"
equation "UpperBodyHeight = 0.8825 in"
equation "WallThickness_Ref = 3.15 mm"
equation "MountingWidthCTC_Ref = 3.75 in"
equation "MountingHeightCTC_Ref = 2.5 in"
equation "MountingDiameter_Ref = ( 7 / 32 ) * 1 in"
equation "MountingDowelThickness_Ref = ( 3 / 64 ) * 1 in"
equation "MountingDowelOutsideDiameter_Ref = MountingDiameter_Ref + ( 2 * MountingDowelThickness_Ref )"
equation "MountingOutsideDiameter_Ref = MountingDowelOutsideDiameter_Ref + ( 2 * WallThickness_Ref )"
equation "MatingHoleWidthCTC_Ref = 4 in"
equation "MatingHoleHeightCTC_Ref = 1 1/4\""
equation "MatingHolePassthroughDiameter_Ref = ( 3 / 16 ) * 1 in"
equation "MatingHoleThreadedDiameter_Ref = ( 1 / 8 ) * 1 in"
equation "MatingHoleSupportDiameter_Ref = ( 1 / 2 ) * 1 in"
equation "BodyBottomDepth_Ref = 1 5/16\""
equation "MountingDowelHeight_Ref = ( 1 / 8 ) * 1 in"
equation "MountingDowelClearance_Ref = 0.01 in"
equation "BearingBoxWidth_Ref = ( 13 / 64 ) * 1 in"
equation "BearingBoxLength_Ref = 0.74 in"
equation "BottomCenterHoleDiameter_Ref = ( 3 / 4 ) * 1 in"
equation "BottomCornerHoleDiameter_Ref = ( 3 / 8 ) * 1 in"
equation "BottomCornerHoleWidthCTC_Ref = 2 11/16\""
equation "BottomCornerHoleHeightCTC_Ref = 1 51/64\""
equation "EncoderArmHeight_Ref = 1 in"
equation "EncoderArmLength_Ref = 1 1/2\""
equation "EncoderArmTriangleBase_Ref = 0.8835 in"
equation "PCBHolderWidth_Ref = ( 5 / 16 ) * 1 in"
equation "PCBHolderHeight_Ref = 1 1/2\""
equation "InsideHeight_Ref = 2.6530 in"
equation "PCBWidth_Ref = 0.0655 in"
equation "PCBHeight_Ref = 1 7/32\""
equation "EncoderArmThickness_Ref = 0.258 in"
equation "EncoderArmInsideThickness_Ref = EncoderArmThickness_Ref - 0.1435 in"
equation "EncoderArmSupportHeight_Ref = 0.9685 in"
equation "LightScrewDistanceToEdgeOfInnerCircle_Ref = 1.1285 in"
equation "LightScrewDiameter_Ref = MatingHoleThreadedDiameter_Ref"
equation "BearinBoxReliefWidth_Ref = ( 5 / 8 ) * 1 in"
equation "BearingBoxReliefHeight_Ref = 0.07 in"
equation "InnerSupportHeight_Ref = 0.6940 in"
equation "InnerSupportLenth_Ref = 1 1/4\""
equation "BearingOD_Ref = ( 5 / 8 ) * 1 in"
equation "BearingChannelDepth_Ref = 0.6255 in"
equation "BearingExtraWidth_Ref = ( 1 / 16 ) * 1 in"
equation "BearingExtraDepth_Ref = ( 1 / 32 ) * 1 in"
equation "ShaftOpeningDiameter_Ref = ( 5 / 16 ) * 1 in"
equation "OutsideSupportOffset_Ref = 0.053 in"
equation "OutsideSupportHeight_Ref = 0.6 in"
equation "d49 = WallThickness_Ref"
equation "d51 = -OutsideSupportHeight"
equation "OutsideSupportHeight = 0.4030 in"
equation "TopOpeningHeight = 2.110 in"
equation "TopOpeningWidth = TopOpeningHeight"
equation "d59 = TopOpeningHeight"
equation "d60 = TopOpeningWidth"
equation "TopOpeningBorder = ( 3 / 16 ) * 1 in"
equation "d62 = TopOpeningBorder"
equation "d63 = -WallThickness_Ref"
equation "d65 = TopOpeningBorderThicknessSides"
equation "d68 = Fillet_Ref"
equation "d70 = Fillet_Ref"
equation "TopOpeningBorderThicknessMiddle = TopOpeningBorderThicknessSides - ( ( 1 / 64 ) * 1 in )"
equation "d72 = TopOpeningBorderThicknessMiddle"
equation "TopOpeningBorderThicknessSides = ( ( 3 / 32 ) * 1 ) * 1 in"
equation "PegOutsideDiameter = 0.1830 in"
equation "d76 = PegOutsideDiameter"
equation "PegDistanceFromEdge = ( ( 0.0955 + 0.2765 ) / 2 ) * 1 in"
equation "d78 = PegDistanceFromEdge"
equation "PinchGuardCircleRadius = 1.025 in + ( PegOutsideDiameter / 2 )"
equation "d80 = PinchGuardCircleRadius * 2"
equation "Fillet_Ref = 0.05 in"
equation "d88 = Fillet_Ref"
equation "PinchGuardInnerLip = 0.1275 in"
equation "d90 = PinchGuardInnerLip"
equation "PinchGuardInnerDepth = ( 5 / 64 ) * 1 in"
equation "d92 = -PinchGuardInnerDepth"
equation "d94 = -PinchGuardInnerDepth"
equation "PegFlapWidth = ( 3 / 4 ) * 1 in"
equation "PegFlapThickness = ( 1 / 8 ) * 1 in"
equation "d98 = PegFlapWidth"
equation "d99 = PegFlapThickness"
equation "d100 = PegFlapWidth"
equation "d101 = PegFlapThickness"
equation "d105 = Fillet_Ref"
equation "InnerPegHoleDiameter = 0.1285 in"
equation "d111 = InnerPegHoleDiameter"
equation "JointCounterboreDiameter = 0.3175 in"
equation "TopCounterboreDiameter = 0.31 in"
equation "CounterboreDepth = 0.160 in"
equation "d117 = JointCounterboreDiameter"
equation "d118 = -CounterboreDepth"
equation "d120 = TopCounterboreDiameter"
equation "d121 = -CounterboreDepth"
equation "d123 = WallThickness_Ref"
equation "d124 = InnerSupportHeight"
equation "InnerSupportHeight = 0.384 in"
equation "d132 = EncoderArmOutsideHeight"
equation "EncoderArmOutsideHeight = 2 in + EncoderArmInsideThickness_Ref"
equation "d135 = -EncoderArmInsideThickness_Ref"
equation "d137 = -EncoderArmThickness_Ref"
equation "UpperEncoderArmSupportHeight = 0.5535 in"
equation "d140 = -UpperEncoderArmSupportHeight"
equation "InnerSupportGap = 0.0175 in"
equation "d147 = InnerSupportGap"
equation "d148 = WallThickness_Ref"
equation "d149 = WallThickness_Ref"
equation "d150 = WallThickness_Ref"
equation "d151 = WallThickness_Ref"
equation "UpperBearingStopLength = ( 3 / 16 ) * 1 in"
equation "d153 = UpperBearingStopLength"
equation "d154 = UpperBearingStopOffset"
equation "UpperBearingStopOffset = ( 1 / 4 ) * 1 in"
equation "d157 = Fillet_Ref"
equation "WallThickness_Ref1 = 3.15 mm"
equation "MountingWidthCTC_Ref1 = 3.75 in"
equation "MountingHeightCTC_Ref1 = 2.5 in"
equation "MountingDiameter_Ref1 = ( 7 / 32 ) * 1 in"
equation "MountingDowelThickness_Ref1 = ( 3 / 64 ) * 1 in"
equation "MountingDowelOutsideDiameter_Ref1 = MountingDiameter_Ref1 + ( 2 * MountingDowelThickness_Ref1 )"
equation "MountingOutsideDiameter_Ref1 = MountingDowelOutsideDiameter_Ref1 + ( 2 * WallThickness_Ref1 )"
equation "MatingHoleWidthCTC_Ref1 = 4 in"
equation "MatingHoleHeightCTC_Ref1 = 1 1/4\""
equation "MatingHolePassthroughDiameter_Ref1 = ( 3 / 16 ) * 1 in"
equation "MatingHoleThreadedDiameter_Ref1 = 0.154 in"
equation "MatingHoleSupportDiameter_Ref1 = ( 1 / 2 ) * 1 in"
equation "BodyBottomDepth_Ref1 = 1 5/16\""
equation "MountingDowelHeight_Ref1 = ( 1 / 8 ) * 1 in"
equation "MountingDowelClearance_Ref1 = 0.01 in"
equation "BearingBoxWidth_Ref1 = ( 13 / 64 ) * 1 in"
equation "BearingBoxLength_Ref1 = 0.74 in"
equation "BottomCenterHoleDiameter_Ref1 = ( 3 / 4 ) * 1 in"
equation "BottomCornerHoleDiameter_Ref1 = ( 3 / 8 ) * 1 in"
equation "BottomCornerHoleWidthCTC_Ref1 = 2 11/16\""
equation "BottomCornerHoleHeightCTC_Ref1 = 1 51/64\""
equation "EncoderArmHeight_Ref1 = 1 in"
equation "EncoderArmLength_Ref1 = 1 1/2\""
equation "EncoderArmTriangleBase_Ref1 = 0.8835 in"
equation "PCBHolderWidth_Ref1 = ( 5 / 16 ) * 1 in"
equation "PCBHolderHeight_Ref1 = 1 1/2\""
equation "InsideHeight_Ref1 = 2.6530 in"
equation "PCBWidth_Ref1 = 0.0655 in"
equation "PCBHeight_Ref1 = 1 7/32\""
equation "EncoderArmThickness_Ref1 = 0.258 in"
equation "EncoderArmInsideThickness_Ref1 = EncoderArmThickness_Ref1 - 0.1435 in"
equation "EncoderArmSupportHeight_Ref1 = 0.9685 in"
equation "LightScrewDistanceToEdgeOfInnerCircle_Ref1 = 1.1285 in"
equation "LightScrewDiameter_Ref1 = 0.113 in"
equation "BearinBoxReliefWidth_Ref1 = ( 5 / 8 ) * 1 in"
equation "BearingBoxReliefHeight_Ref1 = 0.07 in"
equation "InnerSupportHeight_Ref1 = 0.6940 in"
equation "InnerSupportLenth_Ref1 = 1 1/4\""
equation "BearingOD_Ref1 = ( 5 / 8 ) * 1 in"
equation "BearingChannelDepth_Ref1 = 0.6255 in"
equation "BearingExtraWidth_Ref1 = ( 1 / 16 ) * 1 in"
equation "BearingExtraDepth_Ref1 = ( 1 / 32 ) * 1 in"
equation "ShaftOpeningDiameter_Ref1 = ( 5 / 16 ) * 1 in"
equation "OutsideSupportOffset_Ref1 = 0.053 in"
equation "OutsideSupportHeight_Ref1 = 0.6 in"
equation "Fillet_Ref1 = 0.05 in"
equation "d204 = MatingHolePassthroughDiameter_Ref"

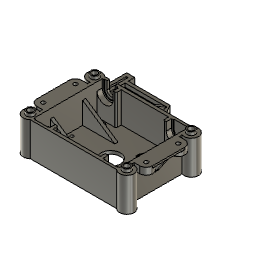
design "039423-01 MH Roller Assembly Bottom"
Autodesk Fusion 360 part; units mm, degrees